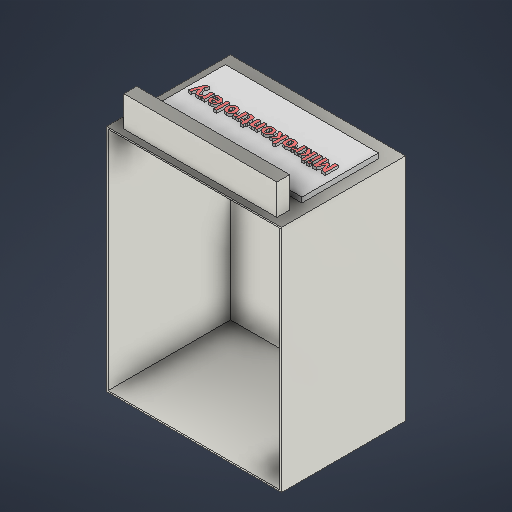
# Autodesk Inventor part: shelf
Saved by Autodesk Inventor 2027 (Build 310192060, 192F)
## iProperties
Created: 2026-06-08
Part Number: shelf
Material: Ogólny
Document SubType Name: Modeling
Designer: User
Density: 1 g/cm^3
Appearance: Domyślna
Author: User
Autodesk Inventor part; units mm, degrees
ref_plane "YZ Plane" through (0, 0, 0) normal (1, 0, 0) x (0, 1, 0)
ref_plane "XZ Plane" through (0, 0, 0) normal (0, 1, 0) x (-1, 0, 0)
ref_plane "XY Plane" through (0, 0, 0) normal (0, 0, 1) x (1, 0, 0)
sketch "Szkic1" plane through (0, 0, 0) normal (0, 1, 0) x (-1, 0, 0)
  line L0 (-34.3, -24.3) -> (34.3, -24.3)
  line L1 (34.3, -24.3) -> (34.3, 24.3)
  line L2 (34.3, 24.3) -> (-34.3, 24.3)
  line L3 (-34.3, 24.3) -> (-34.3, -24.3)
  line L4 (-34.3, -24.3) -> (34.3, 24.3) construction
  line L5 (34.3, -24.3) -> (-34.3, 24.3) construction
  point P0 (0, 0)
  dimension "d0" = 68.6
  dimension "d1" = 48.6
  constraints: 12 end point, 2 midpoint, 2 parallel, 1 horizontal, 1 perpendicular
  measures "d0" distance of L2.end L1.end
  measures "d1" distance of L1.end L0.end
extrude "Wyciągnięcie proste1" add sketch "Szkic1" along normal blind 90
shell "Skorupa1" thickness 0.6 removed faces 1 at (-11.4333, 30, 24.3)
sketch "Szkic2" plane through (0, 90, 0) normal (0, 1, 0) x (1, 0, 0)
  line L0 (-34.3, -24.3) -> (34.3, -24.3) projected
  line L1 (0, -24.3) -> (0, -19.3)
  line L2 (30, -21.8) -> (-30, -21.8)
  line L3 (-30, -21.8) -> (-30, -16.8)
  line L4 (-30, -16.8) -> (30, -16.8)
  line L5 (30, -16.8) -> (30, -21.8)
  line L6 (30, -21.8) -> (-30, -16.8) construction
  line L7 (-30, -21.8) -> (30, -16.8) construction
  point P0 (0, 0)
  dimension "d5" = 5
  dimension "d6" = 60
  dimension "d7" = 5
  constraints: 14 end point, 3 midpoint, 2 parallel, 1 horizontal, 1 perpendicular, 1 vertical
  measures "d5" distance of L1.start L1.end
  measures "d6" distance of L2.start L2.end
  measures "d7" distance of L2.end L3.end
extrude "Wyciągnięcie proste2" add sketch "Szkic2" along normal blind 12
sketch "Szkic3" plane through (0, 90, 0) normal (0, 1, 0) x (1, 0, 0)
  line L0 (0, 0) -> (0, 3)
  line L1 (30, 18) -> (-30, 18)
  line L2 (-30, 18) -> (-30, -12)
  line L3 (-30, -12) -> (30, -12)
  line L4 (30, -12) -> (30, 18)
  line L5 (30, 18) -> (-30, -12) construction
  line L6 (-30, 18) -> (30, -12) construction
  dimension "d10" = 3
  dimension "d11" = 60
  dimension "d12" = 30
  constraints: 14 end point, 2 midpoint, 2 parallel, 1 horizontal, 1 perpendicular, 1 vertical
  measures "d10" distance of L0.start L0.end
  measures "d11" distance of L3.end L2.end
  measures "d12" distance of L2.end L1.end
extrude "Wyciągnięcie proste3" add sketch "Szkic3" along normal blind 2
sketch "Szkic4" plane through (0, 92, 0) normal (0, 1, 0) x (1, 0, 0)
  line L0 (30, -12) -> (-30, -12) construction
  line L1 (-30, -12) -> (-30, 18) construction
  line L2 (-30, 18) -> (30, 18) construction
  line L3 (30, 18) -> (30, -12) construction
  line L4 (-30, -12) -> (30, -12) projected
  line L5 (-30, 18) -> (-30, -12) projected
  line L6 (30, -12) -> (-30, -12)
  line L7 (-30, -12) -> (-30, 18)
  line L8 (-30, 18) -> (30, 18)
  line L9 (30, 18) -> (30, -12)
  line L10 (22.1617, 4.9226) -> (23.4096, 4.9226)
  line L11 (23.4096, 4.9226) -> (23.4096, 1.6082)
  line L12 (23.4096, 1.6082) -> (24.3173, 3.7476)
  line L13 (24.3173, 3.7476) -> (25.1763, 3.7476)
  line L14 (25.1763, 3.7476) -> (26.0839, 1.6082)
  line L15 (26.0839, 1.6082) -> (26.0839, 4.9226)
  line L16 (26.0839, 4.9226) -> (27.267, 4.9226)
  line L17 (27.267, 4.9226) -> (27.267, -0.0774)
  line L18 (27.267, -0.0774) -> (25.8205, -0.0774)
  line L19 (25.8205, -0.0774) -> (24.7103, 2.3902)
  line L20 (24.7103, 2.3902) -> (23.6082, -0.0774)
  line L21 (23.6082, -0.0774) -> (22.1617, -0.0774)
  line L22 (22.1617, -0.0774) -> (22.1617, 4.9226)
  line L23 (20.0182, 4.9226) -> (21.1933, 4.9226)
  line L24 (21.1933, 4.9226) -> (21.1933, 1.1503)
  line L25 (21.1933, 1.1503) -> (20.0182, 1.1503)
  line L26 (20.0182, 1.1503) -> (20.0182, 4.9226)
  line L27 (19.9818, 0.6114) -> (21.2257, 0.6114)
  line L28 (21.2257, 0.6114) -> (21.2257, -0.3043)
  line L29 (21.2257, -0.3043) -> (19.9818, -0.3043)
  line L30 (19.9818, -0.3043) -> (19.9818, 0.6114)
  line L31 (15.3424, 4.9226) -> (16.7403, 4.9226)
  line L32 (16.7403, 4.9226) -> (17.7613, 3.2857)
  line L33 (17.7613, 3.2857) -> (17.9437, 3.5288)
  line L34 (17.9437, 3.5288) -> (17.9437, 4.9226)
  line L35 (17.9437, 4.9226) -> (19.1187, 4.9226)
  line L36 (19.1187, 4.9226) -> (19.1187, -0.3002)
  line L37 (19.1187, -0.3002) -> (17.9437, -0.3002)
  line L38 (17.9437, -0.3002) -> (17.9437, 2.6252)
  line L39 (17.9437, 2.6252) -> (16.8294, 1.1503)
  line L40 (16.8294, 1.1503) -> (15.4396, 1.1503)
  line L41 (15.4396, 1.1503) -> (16.7605, 2.7751)
  line L42 (16.7605, 2.7751) -> (15.3424, 4.9226)
  line L43 (12.4412, 2.2646) -> (12.5385, 2.2646)
  spline S0 degree 2 poles (12.5385, 2.2646) (12.6074, 2.2403) (12.8626, 2.216) (13.0166, 2.216) knots 0 0 0 1 2 2 2
  spline S1 degree 2 poles (13.0166, 2.216) (13.1989, 2.216) (13.6082, 2.3254) (13.7986, 2.3983) knots 0 0 0 1 2 2 2
  line L44 (13.7986, 2.3983) -> (13.7986, 4.9226)
  line L45 (13.7986, 4.9226) -> (14.9737, 4.9226)
  line L46 (14.9737, 4.9226) -> (14.9737, 1.1503)
  line L47 (14.9737, 1.1503) -> (13.7986, 1.1503)
  line L48 (13.7986, 1.1503) -> (13.7986, 1.6933)
  spline S2 degree 2 poles (13.7986, 1.6933) (13.7176, 1.6203) (13.434, 1.3934) (13.3165, 1.3246) knots 0 0 0 1 2 2 2
  spline S3 degree 2 poles (13.3165, 1.3246) (13.1868, 1.2476) (12.8464, 1.1382) (12.6965, 1.1382) knots 0 0 0 1 2 2 2
  spline S4 degree 2 poles (12.6965, 1.1382) (12.6398, 1.1382) (12.498, 1.1463) (12.4412, 1.1503) knots 0 0 0 1 2 2 2
  line L49 (12.4412, 1.1503) -> (12.4412, 2.2646)
  spline S5 degree 2 poles (8.3732, 3.0385) (8.3732, 3.9704) (9.3902, 5.0401) (10.3181, 5.0401) knots 0 0 0 1 2 2 2
  spline S6 degree 2 poles (10.3181, 5.0401) (11.2419, 5.0401) (12.267, 3.9704) (12.267, 3.0385) knots 0 0 0 1 2 2 2
  spline S7 degree 2 poles (12.267, 3.0385) (12.267, 2.0985) (11.2419, 1.0328) (10.3181, 1.0328) knots 0 0 0 1 2 2 2
  spline S8 degree 2 poles (10.3181, 1.0328) (9.3942, 1.0328) (8.3732, 2.1025) (8.3732, 3.0385) knots 0 0 0 1 2 2 2
  spline S9 degree 2 poles (9.5766, 3.0466) (9.5766, 2.7103) (9.686, 2.2605) (9.7832, 2.1268) knots 0 0 0 1 2 2 2
  spline S10 degree 2 poles (9.7832, 2.1268) (9.8886, 1.985) (10.1519, 1.8756) (10.3181, 1.8756) knots 0 0 0 1 2 2 2
  spline S11 degree 2 poles (10.3181, 1.8756) (10.4801, 1.8756) (10.7354, 1.9729) (10.8408, 2.1106) knots 0 0 0 1 2 2 2
  spline S12 degree 2 poles (10.8408, 2.1106) (10.9421, 2.2403) (11.0636, 2.6981) (11.0636, 3.0466) knots 0 0 0 1 2 2 2
  spline S13 degree 2 poles (11.0636, 3.0466) (11.0636, 3.391) (10.9502, 3.8165) (10.857, 3.9461) knots 0 0 0 1 2 2 2
  spline S14 degree 2 poles (10.857, 3.9461) (10.7638, 4.0758) (10.4801, 4.1973) (10.31, 4.1973) knots 0 0 0 1 2 2 2
  spline S15 degree 2 poles (10.31, 4.1973) (10.1682, 4.1973) (9.8764, 4.0758) (9.7873, 3.9542) knots 0 0 0 1 2 2 2
  spline S16 degree 2 poles (9.7873, 3.9542) (9.686, 3.8124) (9.5766, 3.4032) (9.5766, 3.0466) knots 0 0 0 1 2 2 2
  line L50 (3.9729, 4.9226) -> (5.3707, 4.9226)
  line L51 (5.3707, 4.9226) -> (6.3918, 3.2857)
  line L52 (6.3918, 3.2857) -> (6.5741, 3.5288)
  line L53 (6.5741, 3.5288) -> (6.5741, 4.9226)
  line L54 (6.5741, 4.9226) -> (7.7492, 4.9226)
  line L55 (7.7492, 4.9226) -> (7.7492, -0.3002)
  line L56 (7.7492, -0.3002) -> (6.5741, -0.3002)
  line L57 (6.5741, -0.3002) -> (6.5741, 2.6252)
  line L58 (6.5741, 2.6252) -> (5.4599, 1.1503)
  line L59 (5.4599, 1.1503) -> (4.0701, 1.1503)
  line L60 (4.0701, 1.1503) -> (5.391, 2.7751)
  line L61 (5.391, 2.7751) -> (3.9729, 4.9226)
  spline S17 degree 2 poles (-0.0142, 3.0385) (-0.0142, 3.9704) (1.0028, 5.0401) (1.9307, 5.0401) knots 0 0 0 1 2 2 2
  spline S18 degree 2 poles (1.9307, 5.0401) (2.8545, 5.0401) (3.8797, 3.9704) (3.8797, 3.0385) knots 0 0 0 1 2 2 2
  spline S19 degree 2 poles (3.8797, 3.0385) (3.8797, 2.0985) (2.8545, 1.0328) (1.9307, 1.0328) knots 0 0 0 1 2 2 2
  spline S20 degree 2 poles (1.9307, 1.0328) (1.0069, 1.0328) (-0.0142, 2.1025) (-0.0142, 3.0385) knots 0 0 0 1 2 2 2
  spline S21 degree 2 poles (1.1892, 3.0466) (1.1892, 2.7103) (1.2986, 2.2605) (1.3959, 2.1268) knots 0 0 0 1 2 2 2
  spline S22 degree 2 poles (1.3959, 2.1268) (1.5012, 1.985) (1.7646, 1.8756) (1.9307, 1.8756) knots 0 0 0 1 2 2 2
  spline S23 degree 2 poles (1.9307, 1.8756) (2.0928, 1.8756) (2.3481, 1.9729) (2.4534, 2.1106) knots 0 0 0 1 2 2 2
  spline S24 degree 2 poles (2.4534, 2.1106) (2.5547, 2.2403) (2.6763, 2.6981) (2.6763, 3.0466) knots 0 0 0 1 2 2 2
  spline S25 degree 2 poles (2.6763, 3.0466) (2.6763, 3.391) (2.5628, 3.8165) (2.4696, 3.9461) knots 0 0 0 1 2 2 2
  spline S26 degree 2 poles (2.4696, 3.9461) (2.3764, 4.0758) (2.0928, 4.1973) (1.9226, 4.1973) knots 0 0 0 1 2 2 2
  spline S27 degree 2 poles (1.9226, 4.1973) (1.7808, 4.1973) (1.4891, 4.0758) (1.3999, 3.9542) knots 0 0 0 1 2 2 2
  spline S28 degree 2 poles (1.3999, 3.9542) (1.2986, 3.8124) (1.1892, 3.4032) (1.1892, 3.0466) knots 0 0 0 1 2 2 2
  line L62 (-4.1673, 4.9226) -> (-2.9842, 4.9226)
  line L63 (-2.9842, 4.9226) -> (-2.9842, 3.0547)
  spline S29 degree 2 poles (-2.9842, 3.0547) (-2.9842, 2.8237) (-2.9477, 2.3699) (-2.8991, 2.2646) knots 0 0 0 1 2 2 2
  spline S30 degree 2 poles (-2.8991, 2.2646) (-2.8383, 2.1349) (-2.6114, 2.0255) (-2.4169, 2.0255) knots 0 0 0 1 2 2 2
  spline S31 degree 2 poles (-2.4169, 2.0255) (-2.2751, 2.0255) (-1.9793, 2.1349) (-1.8132, 2.2524) knots 0 0 0 1 2 2 2
  line L64 (-1.8132, 2.2524) -> (-1.8132, 4.9226)
  line L65 (-1.8132, 4.9226) -> (-0.6382, 4.9226)
  line L66 (-0.6382, 4.9226) -> (-0.6382, 1.1503)
  line L67 (-0.6382, 1.1503) -> (-1.8132, 1.1503)
  line L68 (-1.8132, 1.1503) -> (-1.8132, 1.5677)
  spline S32 degree 2 poles (-1.8132, 1.5677) (-2.1009, 1.3246) (-2.6479, 1.049) (-2.9801, 1.049) knots 0 0 0 1 2 2 2
  spline S33 degree 2 poles (-2.9801, 1.049) (-3.5555, 1.049) (-4.1673, 1.7784) (-4.1673, 2.4672) knots 0 0 0 1 2 2 2
  line L69 (-4.1673, 2.4672) -> (-4.1673, 4.9226)
  spline S34 degree 2 poles (-6.481, 4.9955) (-5.7638, 4.9955) (-5.1074, 4.404) (-5.1074, 3.7314) knots 0 0 0 1 2 2 2
  line L70 (-5.1074, 3.7314) -> (-5.1074, 1.9688)
  line L71 (-5.1074, 1.9688) -> (-4.6576, 1.9688)
  line L72 (-4.6576, 1.9688) -> (-4.6576, 1.1503)
  line L73 (-4.6576, 1.1503) -> (-5.1074, 1.1503)
  line L74 (-5.1074, 1.1503) -> (-5.1074, 0.0725)
  line L75 (-5.1074, 0.0725) -> (-6.2824, 0.0725)
  line L76 (-6.2824, 0.0725) -> (-6.2824, 1.1503)
  line L77 (-6.2824, 1.1503) -> (-7.4169, 1.1503)
  line L78 (-7.4169, 1.1503) -> (-7.4169, 1.9688)
  line L79 (-7.4169, 1.9688) -> (-6.2824, 1.9688)
  line L80 (-6.2824, 1.9688) -> (-6.2824, 3.31)
  spline S35 degree 2 poles (-6.2824, 3.31) (-6.2824, 3.5085) (-6.2905, 3.8043) (-6.3391, 3.9218) knots 0 0 0 1 2 2 2
  spline S36 degree 2 poles (-6.3391, 3.9218) (-6.3878, 4.0393) (-6.6268, 4.1771) (-6.8537, 4.1771) knots 0 0 0 1 2 2 2
  spline S37 degree 2 poles (-6.8537, 4.1771) (-6.951, 4.1771) (-7.2549, 4.096) (-7.3156, 4.0636) knots 0 0 0 1 2 2 2
  line L81 (-7.3156, 4.0636) -> (-7.4169, 4.0636)
  line L82 (-7.4169, 4.0636) -> (-7.4169, 4.8902)
  spline S38 degree 2 poles (-7.4169, 4.8902) (-7.2265, 4.9388) (-6.797, 4.9955) (-6.481, 4.9955) knots 0 0 0 1 2 2 2
  line L83 (-10.4275, 2.2646) -> (-10.3302, 2.2646)
  spline S39 degree 2 poles (-10.3302, 2.2646) (-10.2613, 2.2403) (-10.0061, 2.216) (-9.8521, 2.216) knots 0 0 0 1 2 2 2
  spline S40 degree 2 poles (-9.8521, 2.216) (-9.6698, 2.216) (-9.2605, 2.3254) (-9.0701, 2.3983) knots 0 0 0 1 2 2 2
  line L84 (-9.0701, 2.3983) -> (-9.0701, 4.9226)
  line L85 (-9.0701, 4.9226) -> (-7.8951, 4.9226)
  line L86 (-7.8951, 4.9226) -> (-7.8951, 1.1503)
  line L87 (-7.8951, 1.1503) -> (-9.0701, 1.1503)
  line L88 (-9.0701, 1.1503) -> (-9.0701, 1.6933)
  spline S41 degree 2 poles (-9.0701, 1.6933) (-9.1511, 1.6203) (-9.4348, 1.3934) (-9.5523, 1.3246) knots 0 0 0 1 2 2 2
  spline S42 degree 2 poles (-9.5523, 1.3246) (-9.6819, 1.2476) (-10.0223, 1.1382) (-10.1722, 1.1382) knots 0 0 0 1 2 2 2
  spline S43 degree 2 poles (-10.1722, 1.1382) (-10.2289, 1.1382) (-10.3707, 1.1463) (-10.4275, 1.1503) knots 0 0 0 1 2 2 2
  line L89 (-10.4275, 1.1503) -> (-10.4275, 2.2646)
  spline S44 degree 2 poles (-14.4955, 3.0385) (-14.4955, 3.9704) (-13.4785, 5.0401) (-12.5506, 5.0401) knots 0 0 0 1 2 2 2
  spline S45 degree 2 poles (-12.5506, 5.0401) (-11.6268, 5.0401) (-10.6017, 3.9704) (-10.6017, 3.0385) knots 0 0 0 1 2 2 2
  spline S46 degree 2 poles (-10.6017, 3.0385) (-10.6017, 2.0985) (-11.6268, 1.0328) (-12.5506, 1.0328) knots 0 0 0 1 2 2 2
  spline S47 degree 2 poles (-12.5506, 1.0328) (-13.4745, 1.0328) (-14.4955, 2.1025) (-14.4955, 3.0385) knots 0 0 0 1 2 2 2
  spline S48 degree 2 poles (-13.2921, 3.0466) (-13.2921, 2.7103) (-13.1827, 2.2605) (-13.0855, 2.1268) knots 0 0 0 1 2 2 2
  spline S49 degree 2 poles (-13.0855, 2.1268) (-12.9801, 1.985) (-12.7168, 1.8756) (-12.5506, 1.8756) knots 0 0 0 1 2 2 2
  spline S50 degree 2 poles (-12.5506, 1.8756) (-12.3886, 1.8756) (-12.1333, 1.9729) (-12.028, 2.1106) knots 0 0 0 1 2 2 2
  spline S51 degree 2 poles (-12.028, 2.1106) (-11.9267, 2.2403) (-11.8051, 2.6981) (-11.8051, 3.0466) knots 0 0 0 1 2 2 2
  spline S52 degree 2 poles (-11.8051, 3.0466) (-11.8051, 3.391) (-11.9186, 3.8165) (-12.0118, 3.9461) knots 0 0 0 1 2 2 2
  spline S53 degree 2 poles (-12.0118, 3.9461) (-12.1049, 4.0758) (-12.3886, 4.1973) (-12.5588, 4.1973) knots 0 0 0 1 2 2 2
  spline S54 degree 2 poles (-12.5588, 4.1973) (-12.7006, 4.1973) (-12.9923, 4.0758) (-13.0814, 3.9542) knots 0 0 0 1 2 2 2
  spline S55 degree 2 poles (-13.0814, 3.9542) (-13.1827, 3.8124) (-13.2921, 3.4032) (-13.2921, 3.0466) knots 0 0 0 1 2 2 2
  line L90 (-16.2946, 4.9226) -> (-15.1195, 4.9226)
  line L91 (-15.1195, 4.9226) -> (-15.1195, -0.3002)
  line L92 (-15.1195, -0.3002) -> (-16.2946, -0.3002)
  line L93 (-16.2946, -0.3002) -> (-16.2946, 4.9226)
  spline S56 degree 2 poles (-19.1268, 5.0239) (-18.0571, 5.0239) (-16.9186, 4.0028) (-16.9186, 3.0588) knots 0 0 0 1 2 2 2
  spline S57 degree 2 poles (-16.9186, 3.0588) (-16.9186, 2.1349) (-17.9801, 1.0328) (-18.9364, 1.0328) knots 0 0 0 1 2 2 2
  spline S58 degree 2 poles (-18.9364, 1.0328) (-19.7994, 1.0328) (-20.6746, 1.9688) (-20.6746, 2.8359) knots 0 0 0 1 2 2 2
  line L94 (-20.6746, 2.8359) -> (-20.6746, 3.2613)
  line L95 (-20.6746, 3.2613) -> (-18.0936, 3.2613)
  spline S59 degree 2 poles (-18.0936, 3.2613) (-18.1098, 3.5247) (-18.3002, 3.8732) (-18.4542, 3.9785) knots 0 0 0 1 2 2 2
  spline S60 degree 2 poles (-18.4542, 3.9785) (-18.6041, 4.0839) (-19.0093, 4.173) (-19.2484, 4.173) knots 0 0 0 1 2 2 2
  spline S61 degree 2 poles (-19.2484, 4.173) (-19.451, 4.173) (-19.8481, 4.0839) (-20.0142, 4.0069) knots 0 0 0 1 2 2 2
  spline S62 degree 2 poles (-20.0142, 4.0069) (-20.16, 3.9461) (-20.4032, 3.7962) (-20.4801, 3.7395) knots 0 0 0 1 2 2 2
  line L96 (-20.4801, 3.7395) -> (-20.6058, 3.7395)
  line L97 (-20.6058, 3.7395) -> (-20.6058, 4.7119)
  spline S63 degree 2 poles (-20.6058, 4.7119) (-20.4599, 4.7686) (-20.2249, 4.8659) (-20.0142, 4.9145) knots 0 0 0 1 2 2 2
  spline S64 degree 2 poles (-20.0142, 4.9145) (-19.8237, 4.9672) (-19.4186, 5.0239) (-19.1268, 5.0239) knots 0 0 0 1 2 2 2
  spline S65 degree 2 poles (-19.5158, 2.5523) (-19.5077, 2.1795) (-19.1795, 1.7865) (-18.8432, 1.7865) knots 0 0 0 1 2 2 2
  spline S66 degree 2 poles (-18.8432, 1.7865) (-18.4988, 1.7865) (-18.1098, 2.1998) (-18.0895, 2.5523) knots 0 0 0 1 2 2 2
  line L98 (-18.0895, 2.5523) -> (-19.5158, 2.5523)
  line L99 (-23.8108, 2.2646) -> (-23.7135, 2.2646)
  spline S67 degree 2 poles (-23.7135, 2.2646) (-23.6447, 2.2403) (-23.3894, 2.216) (-23.2354, 2.216) knots 0 0 0 1 2 2 2
  spline S68 degree 2 poles (-23.2354, 2.216) (-23.0531, 2.216) (-22.6438, 2.3254) (-22.4534, 2.3983) knots 0 0 0 1 2 2 2
  line L100 (-22.4534, 2.3983) -> (-22.4534, 4.9226)
  line L101 (-22.4534, 4.9226) -> (-21.2784, 4.9226)
  line L102 (-21.2784, 4.9226) -> (-21.2784, 1.1503)
  line L103 (-21.2784, 1.1503) -> (-22.4534, 1.1503)
  line L104 (-22.4534, 1.1503) -> (-22.4534, 1.6933)
  spline S69 degree 2 poles (-22.4534, 1.6933) (-22.5344, 1.6203) (-22.8181, 1.3934) (-22.9356, 1.3246) knots 0 0 0 1 2 2 2
  spline S70 degree 2 poles (-22.9356, 1.3246) (-23.0652, 1.2476) (-23.4056, 1.1382) (-23.5555, 1.1382) knots 0 0 0 1 2 2 2
  spline S71 degree 2 poles (-23.5555, 1.1382) (-23.6122, 1.1382) (-23.7541, 1.1463) (-23.8108, 1.1503) knots 0 0 0 1 2 2 2
  line L105 (-23.8108, 1.1503) -> (-23.8108, 2.2646)
  line L106 (-27.7776, 1.1503) -> (-25.8772, 6.3043)
  line L107 (-25.8772, 6.3043) -> (-24.613, 6.3043)
  line L108 (-24.613, 6.3043) -> (-25.1844, 4.8294)
  line L109 (-25.1844, 4.8294) -> (-23.8027, 1.1503)
  line L110 (-23.8027, 1.1503) -> (-25.0344, 1.1503)
  line L111 (-25.0344, 1.1503) -> (-25.8286, 3.5166)
  line L112 (-25.8286, 3.5166) -> (-26.5701, 1.1503)
  line L113 (-26.5701, 1.1503) -> (-27.7776, 1.1503)
  point P0 (0, 0)
  dimension "d0" = 68.6
  dimension "d1" = 48.6
  constraints: 8 end point, 2 coincident, 2 parallel, 1 horizontal, 1 perpendicular, 2 other
extrude "Wyciągnięcie proste4" add sketch "Szkic4" along normal blind 1 contours L10 L11 L12 L13 L14 L15 L16 L17 L18 L19 L20 L21 L22 | L23 L24 L25 L26 | L27 L28 L29 L30 | L31 L32 L33 L34 L35 L36 L37 L38 L39 L40 L41 L42 | L43 S0 S1 L44 L45 L46 L47 L48 S2 S3 S4 L49 | S5 S6 S7 S8 | L50 L51 L52 L53 L54 L55 L56 L57 L58 L59 L60 L61 | S17 S18 S19 S20 | L62 L63 S29 S30 S31 L64 L65 L66 L67 L68 S32 S33 L69 | S34 L70 L71 L72 L73 L74 L75 L76 L77 L78 L79 L80 S35 S36 S37 L81 L82 S38 | L83 S39 S40 L84 L85 L86 L87 L88 S41 S42 S43 L89 | S44 S45 S46 S47 | L90 L91 L92 L93 | S56 S57 S58 L94 L95 S59 S60 S61 S62 L96 L97 S63 S64 | L99 S67 S68 L100 L101 L102 L103 L104 S69 S70 S71 L109 L105 | L109 S71 L105 | L105 L110 L111 L112 L113 L106 L107 L108 L109
